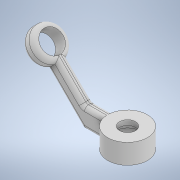
# Autodesk Inventor part: Skrzynia-srodek-ramie
Saved by Autodesk Inventor 2022 (Build 260153000, 153)
## iProperties
Created: 2022-03-27
Part Number: Skrzynia-srodek-ramie
Material: Ogólny
Document SubType Name: Modeling
Designer: jolow
Density: 1 g/cm^3
Appearance: Domyślna
Author: jolow
Autodesk Inventor part; units mm, degrees
ref_plane "YZ Plane" through (0, 0, 0) normal (1, 0, 0) x (0, 1, 0)
ref_plane "XZ Plane" through (0, 0, 0) normal (0, 1, 0) x (-1, 0, 0)
ref_plane "XY Plane" through (0, 0, 0) normal (0, 0, 1) x (1, 0, 0)
sketch "Szkic1" plane through (0, 0, 0) normal (0, 1, 0) x (-1, 0, 0)
  circle A0 centre (0, 0) radius 20
  dimension "d0" = 40
  constraints: 1 centre point, 1 coincident
  measures "d0" diameter of A0
extrude "Wyciągnięcie proste1" add sketch "Szkic1" along normal mid plane 20
sketch "Szkic3" plane through (0, 0, 0) normal (0, 0, 1) x (1, 0, 0)
  line L0 (-20, -10) -> (20, -10) projected
  line L1 (0, -10) -> (-40, -10)
  line L2 (-40, -10) -> (-40, 10)
  line L3 (-40, 10) -> (0, 10)
  line L4 (0, 10) -> (0, -10)
  line L5 (-40, 10) -> (-76, 46)
  line L6 (-76, 46) -> (-86, 36)
  line L7 (-86, 36) -> (-40, -10)
  line L8 (0, 10) -> (0, 122)
  line L9 (0, 122) -> (-76, 46)
  point P0 (0, 0)
  dimension "d6" = 45
  dimension "d7" = 112
  dimension "d8" = 20
  dimension "d9" = 40
  dimension "d33" = 107.4802
  constraints: 18 end point, 3 parallel, 3 perpendicular, 1 horizontal, 1 midpoint, 1 vertical
  measures "d6" angle of L9 L8
  measures "d7" distance of L3.end L8.end
  measures "d8" distance of L1.end L2.end
  measures "d9" distance of L2.end L3.end
  measures "d33" distance of L8.end L5.end
extrude "Wyciągnięcie proste3" add sketch "Szkic3" along normal mid plane 10 contours L1 L2 L3 L4 L0 | L7 L6 L5 L2
sketch "Szkic4" plane through (-76, 46, -5) normal (0.7071068, 0.7071068, 0) x (-0.7071068, 0.7071068, 0)
  line L0 (0, 0) -> (0, 10) projected
  circle A0 centre (0, 5) radius 11
  circle A1 centre (0, 5) radius 16
  point P0 (-86.267, 5)
  dimension "d12" = 22
  dimension "d13" = 5
  constraints: 2 centre point, 1 coincident, 1 midpoint
  measures "d12" diameter of A0
  measures "d13" radial gap between concentric circles of A1 A0
extrude "Wyciągnięcie proste4" add sketch "Szkic4" against normal up to surface (14.1421 mm away)
sketch "Szkic5" plane through (-40, 10, -5) normal (0.7071068, 0.7071068, 0) x (-0.7071068, 0.7071068, 0)
  line L0 (50.9117, 0) -> (50.9117, 10) projected
  circle A0 centre (50.9117, 5) radius 11
  point P0 (-35.3553, 5)
  constraints: 1 centre point, 1 midpoint
extrude "Wyciągnięcie proste5" cut sketch "Szkic5" against normal through all
fillet "Zaokrąglenie1" radius 4 11 edges at (-29.6825, 10, -5) (-29.6825, 10, 5) (-52.6265, 22.6265, -5) (-52.6265, 22.6265, 5) (-29.6825, -10, -5) (-29.6825, -10, 5) (-40, -10, 0) (-57.6265, 7.6265, -5) (-57.6265, 7.6265, 5) (-40, 10, 0) (-97.3137, 47.3137, 0)
sketch "Szkic7" plane through (0, -10, 0) normal (0, -1, 0) x (1, 0, 0)
  circle A0 centre (0, 0) radius 15
  dimension "d22" = 30
  constraints: 1 centre point, 1 coincident
  measures "d22" diameter of A0
extrude "Wyciągnięcie proste7" cut sketch "Szkic7" against normal through all
sketch "Szkic8" plane through (0, 10, 0) normal (0, 1, 0) x (1, 0, 0)
  circle A0 centre (0, 0) radius 15
  constraints: 1 centre point, 1 coincident
extrude "Wyciągnięcie proste8" add sketch "Szkic8" against normal blind 10
sketch "Szkic9" plane through (0, 0, 0) normal (0, -1, 0) x (1, 0, 0)
  circle A0 centre (0, 0) radius 8
  dimension "d27" = 16
  constraints: 1 centre point, 1 coincident
  measures "d27" diameter of A0
extrude "Wyciągnięcie proste9" cut sketch "Szkic9" against normal blind 10
sketch "Szkic10" plane through (0, 0, 0) normal (0, -1, 0) x (1, 0, 0)
  circle A0 centre (0, 0) radius 12
  circle A1 centre (0, 0) radius 8.8235
  dimension "d30" = 24
  constraints: 2 centre point, 2 coincident
  measures "d30" diameter of A0
extrude "Wyciągnięcie proste10" cut sketch "Szkic10" against normal blind 5 contours A0 | A1
fillet "Zaokrąglenie2" radius 5 1 edges at (-87.3137, 57.3137, 0)
